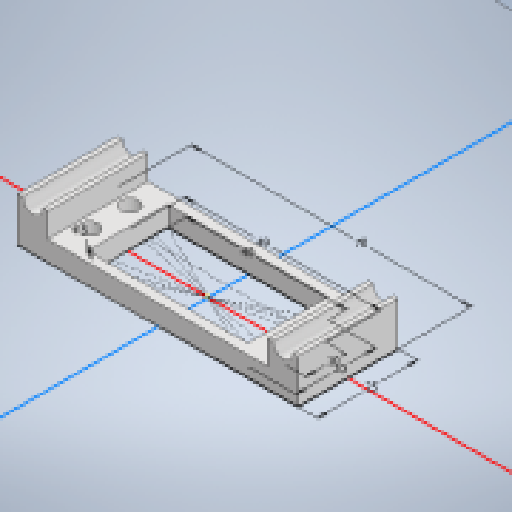
# Autodesk Inventor part: Servo mount
Saved by Autodesk Inventor 2025.2 (Build 292293000, 293)
## iProperties
Created: 2025-01-10
Part Number: Servo mount
Material: Generic
Document SubType Name: Modeling
Designer: caomi
Density: 1 g/cm^3
Appearance: Default
Author: caomi
Autodesk Inventor part; units mm, degrees
ref_plane "YZ Plane" through (0, 0, 0) normal (1, 0, 0) x (0, 1, 0)
ref_plane "XZ Plane" through (0, 0, 0) normal (0, 1, 0) x (-1, 0, 0)
ref_plane "XY Plane" through (0, 0, 0) normal (0, 0, 1) x (1, 0, 0)
sketch "Sketch1" plane through (0, 0, 0) normal (0, 1, 0) x (-1, 0, 0)
  line L0 (-35, -12.5) -> (35, -12.5)
  line L1 (35, -12.5) -> (35, 12.5)
  line L2 (35, 12.5) -> (-35, 12.5)
  line L3 (-35, 12.5) -> (-35, -12.5)
  line L4 (-35, -12.5) -> (35, 12.5) construction
  line L5 (35, -12.5) -> (-35, 12.5) construction
  line L6 (-24.5, -5) -> (24.5, -5) construction
  line L7 (24.5, -5) -> (24.5, 5) construction
  line L8 (24.5, 5) -> (-24.5, 5) construction
  line L9 (-24.5, 5) -> (-24.5, -5) construction
  line L10 (-24.5, -5) -> (24.5, 5) construction
  line L11 (24.5, -5) -> (-24.5, 5) construction
  circle A0 centre (24.5, 5) radius 2.25
  circle A1 centre (24.5, -5) radius 2.25
  circle A2 centre (-24.5, -5) radius 2.25
  circle A3 centre (-24.5, 5) radius 2.25
  line L12 (-20, -10) -> (20, -10)
  line L13 (20, -10) -> (20, 10)
  line L14 (20, 10) -> (-20, 10)
  line L15 (-20, 10) -> (-20, -10)
  line L16 (-20, -10) -> (20, 10) construction
  line L17 (20, -10) -> (-20, 10) construction
  point P0 (0, 0)
  dimension "d0" = 10
  dimension "d1" = 49
  dimension "d2" = 4.5
  dimension "d5" = 25
  dimension "d6" = 70
  dimension "d7" = 20
  dimension "d8" = 40
  constraints: 36 end point, 6 midpoint, 6 parallel, 4 centre point, 4 coincident, 3 equal radius, 3 horizontal, 3 perpendicular
  measures "d0" distance of L8.end L6.start
  measures "d1" distance of L6.start L6.end
  measures "d2" diameter of A0
  measures "d5" distance of L2.end L0.start
  measures "d6" distance of L0.start L0.end
  measures "d7" distance of L14.end L12.start
  measures "d8" distance of L12.start L12.end
extrude "Extrusion1" add sketch "Sketch1" along normal blind 5
sketch "Sketch2" plane through (35, 0, -12.5) normal (0, 0, -1) x (-1, 0, 0)
  line L0 (62.5, 5) -> (62.5, 11)
  line L1 (62.5, 11) -> (70, 11)
  line L2 (70, 11) -> (70, 5)
  line L3 (70, 5) -> (62.5, 5)
  line L4 (35, -3.7897) -> (35, 10.3895) construction
  circle A0 centre (66.25, 11) radius 2.5
  line L5 (0, 5) -> (7.5, 5)
  circle A1 centre (66.25, 11) radius 2.3
  line L6 (7.5, 5) -> (7.5, 11)
  line L7 (7.5, 11) -> (0, 11)
  line L8 (0, 11) -> (0, 5)
  line L9 (0, 5) -> (7.5, 5)
  circle A2 centre (3.75, 11) radius 2.5
  circle A3 centre (3.75, 11) radius 2.3
  line L10 (0, 0) -> (70, 0) projected
  point P0 (35, 0)
  point P1 (35, 0)
  point P2 (68.75, 11)
  point P3 (63.75, 11)
  point P4 (35, 0)
  point P5 (6.05, 11)
  point P6 (1.45, 11)
  point P7 (1.25, 11)
  point P8 (6.25, 11)
  point P9 (68.55, 11)
  point P10 (63.95, 11)
  dimension "d9" = 5
  dimension "d10" = 7.5
  dimension "d12" = 6
  dimension "d18" = 0.2
  constraints: 20 end point, 5 symmetric about line, 4 centre point, 3 perpendicular, 2 midpoint, 2 point on line, 2 vertical, 1 coincident, 2 other
  measures "d9" diameter of A0
  measures "d10" distance of L0.end L1.end
  measures "d12" distance of L1.end L2.end
  measures "d18" radial gap between concentric circles of A1 A0
extrude "Extrusion2" add sketch "Sketch2" against normal up to surface (25 mm away) contours L0 L1 A0 L2 L3 | L8 L7 A2 L6 L5
extrude "Extrusion4" add sketch "Sketch2" against normal blind 2 contours L1 A1 A0 | L7 A3 A2 picked at (64.2095, 9.7038) picked at (6.1368, 10.6171)
mirror "Mirror1" about plane through (0, 0, 0) normal (0, 0, 1) of "Extrusion4"
body "Solid1"
